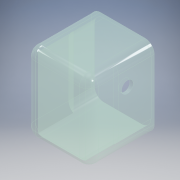
# Autodesk Inventor part: Case_Top
Saved by Autodesk Inventor 2020 (Build 240168000, 168)
## iProperties
Created: 2020-02-24
Part Number: Case_Top
Material: 일반
Document SubType Name: Modeling
Designer: Knowblesse
Density: 1 g/cm^3
Appearance: 기본값
Author: Knowblesse
## iProperties of the stored document _3D 인쇄.ipt
Created: 2020-04-09
Part Number: _3D 인쇄
Material: 일반
Document SubType Name: Modeling
Designer: Knowblesse
Density: 1 g/cm^3
Appearance: 기본값
Author: Knowblesse
Autodesk Inventor part; units mm, degrees
ref_plane "YZ Plane" through (0, 0, 0) normal (1, 0, 0) x (0, 1, 0)
ref_plane "XZ Plane" through (0, 0, 0) normal (0, 1, 0) x (-1, 0, 0)
ref_plane "XY Plane" through (0, 0, 0) normal (0, 0, 1) x (1, 0, 0)
sketch "스케치1" plane through (0, 0, 0) normal (0, 0, 1) x (1, 0, 0)
  line L0 (0, 0) -> (12.1, 0)
  line L1 (12.1, 0) -> (12.1, 15.6)
  line L2 (12.1, 15.6) -> (0, 15.6)
  line L3 (0, 15.6) -> (0, 0)
  line L4 (-0.7, 16.3) -> (12.8, 16.3)
  line L5 (12.8, 16.3) -> (12.8, -0.7)
  line L6 (12.8, -0.7) -> (-0.7, -0.7)
  line L7 (-0.7, -0.7) -> (-0.7, 16.3)
  dimension "d0" = 12.1
  dimension "d1" = 15.6
  dimension "d2" = 0.7
  constraints: 16 end point, 4 parallel, 2 perpendicular, 1 horizontal, 3 other
  measures "d0" distance of L1.end L2.end
  measures "d1" distance between parallel lines of L0 L2
  measures "d2" distance between parallel lines of L2 L4
extrude "돌출1" add sketch "스케치1" along normal blind 7
sketch "스케치2" plane through (0, 0, 7) normal (0, 0, 1) x (1, 0, 0)
  line L0 (-0.7, 16.3) -> (-0.7, -0.7) projected
  line L1 (-0.7, -0.7) -> (12.8, -0.7) projected
  line L2 (12.8, -0.7) -> (12.8, 16.3) projected
  line L3 (12.8, 16.3) -> (-0.7, 16.3) projected
  line L4 (12.1, 0) -> (0, 0) projected
  line L5 (0, 0) -> (0, 15.6) projected
  line L6 (0, 15.6) -> (12.1, 15.6) projected
  line L7 (12.1, 15.6) -> (12.1, 0) projected
  line L8 (1, 15.6) -> (1, 0)
  line L9 (12.1, 0) -> (0, 0) projected
  line L10 (11.1, 15.6) -> (11.1, 0)
  line L11 (0, 15.6) -> (12.1, 15.6) projected
  dimension "d5" = 1
  dimension "d6" = 1
  constraints: 4 end point, 4 point on line, 2 perpendicular
  measures "d5" distance between parallel lines of L5 L8
  measures "d6" distance between parallel lines of L7 L10
extrude "돌출2" add sketch "스케치2" along normal blind 6 contours L3 L2 L1 L0 | L4 L10 L6 L7 | L4 L5 L6 L8
fillet "모깎기1" radius 2 4 edges at (0, 15.6, 3.5) (12.1, 15.6, 3.5) (12.1, 0, 3.5) (0, 0, 3.5)
sketch "스케치3" plane through (0, 0, 13) normal (0, 0, 1) x (1, 0, 0)
  line L0 (-0.7, -0.7) -> (12.8, -0.7) projected
  line L1 (12.8, -0.7) -> (12.8, 16.3) projected
  line L2 (12.8, 16.3) -> (-0.7, 16.3) projected
  line L3 (-0.7, 16.3) -> (-0.7, -0.7) projected
  line L4 (10.1, 0) -> (2, 0) projected
  arc A0 (1, 0.2679) -> (2, 0) centre (2, 2) ccw projected
  line L5 (1, 0.2679) -> (1, 15.3321) projected
  arc A1 (2, 15.6) -> (1, 15.3321) centre (2, 13.6) ccw projected
  line L6 (2, 15.6) -> (10.1, 15.6) projected
  arc A2 (11.1, 15.3321) -> (10.1, 15.6) centre (10.1, 13.6) ccw projected
  line L7 (11.1, 15.3321) -> (11.1, 0.2679) projected
  arc A3 (10.1, 0) -> (11.1, 0.2679) centre (10.1, 2) ccw projected
  point P0 (0, 0)
extrude "돌출3" add sketch "스케치3" along normal blind 1 contours L3 L2 L1 L0 | L4 A0 L5 A1 L6 A2 L7 A3
sketch "스케치4" plane through (12.8, -0.7, 0) normal (1, 0, 0) x (0, 0, -1)
  line L0 (-7, 14.3) -> (-7, 2.7) projected
  line L1 (-13, 16.3) -> (0, 16.3) projected
  point P0 (0, 0.7)
  point P1 (-5.75, 11.8)
  dimension "d12" = 1.25
  dimension "d14" = 4.5
  measures "d12" distance from line of L0 point (-5.75, 11.8)
  measures "d14" distance from line of L1 point (-5.75, 11.8)
hole "구멍1" at (12.8, 11.1, 5.75) direction (-1, 0, 0) diameter 2.5 depth 0.7 tip angle 118
fillet "모깎기2" radius 2 8 edges at (12.8, -0.7, 7) (-0.7, -0.7, 7) (12.8, 16.3, 7) (-0.7, 16.3, 7) (12.8, 7.8, 14) (6.05, -0.7, 14) (-0.7, 7.8, 14) (6.05, 16.3, 14)
sketch "스케치5" plane through (0, 0, 7) normal (0, 0, -1) x (-1, 0, 0)
  arc A0 (-1, 0.2679) -> (0, 2) centre (-2, 2) ccw projected
  line L0 (0, 2) -> (0, 13.6) projected
  arc A1 (0, 13.6) -> (-1, 15.3321) centre (-2, 13.6) ccw projected
  line L1 (-1, 0.2679) -> (-1, 15.3321) projected
  point P0 (0, 0)
extrude "돌출4" add sketch "스케치5" along normal blind 1.5
